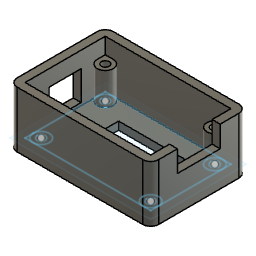
usb2uart (Autodesk Fusion 360 design; units mm, degrees)
Autodesk Fusion 360 part; units mm, degrees
sketch "Sketch1" plane through (0, 0, 0) normal (0, 1, 0) x (1, 0, 0)
  line L0 (0, 0) -> (53, 0)
  line L1 (53, 0) -> (53, -36)
  line L2 (53, -36) -> (0, -36)
  line L3 (0, -36) -> (0, 0)
  constraint horizontal L0
  constraint vertical L1
  constraint horizontal L2
  constraint vertical L3
  constraint coincident L0.start L3.end
extrude "Extrude1" add sketch "Sketch1" along normal blind 3
sketch "Sketch2" plane through (0, 3, 0) normal (0, 1, 0) x (-1, 0, 0)
  line L0 (0, 36) -> (-53, 36)
  line L1 (-53, 36) -> (-53, 0)
  line L2 (-53, 0) -> (0, 0)
  line L3 (0, 0) -> (0, 36)
  line L4 (-3, 3) -> (-50, 3)
  line L5 (-50, 3) -> (-50, 33)
  line L6 (-50, 33) -> (-3, 33)
  line L7 (-3, 33) -> (-3, 3)
  circle A0 centre (-47, 30) radius 3
  circle A1 centre (-47, 6) radius 3
  circle A2 centre (-6, 30) radius 3
  circle A3 centre (-6, 6) radius 3
  circle A4 centre (-6, 6) radius 1.5
  circle A5 centre (-6, 30) radius 1.5
  circle A6 centre (-47, 30) radius 1.5
  circle A7 centre (-47, 6) radius 1.5
  dimension "d3" = 6
  dimension "d4" = 6
  dimension "d5" = 3
  dimension "d6" = 3
  dimension "d7" = 3
  constraint horizontal L4
  constraint vertical L5
  constraint horizontal L6
  constraint vertical L7
  constraint tangent L7 A2
  constraint tangent L7 A3
  constraint concentric A3 A4
  constraint concentric A2 A5
  constraint concentric A0 A6
  constraint concentric A1 A7
  measures "d3" diameter of A1
  measures "d4" diameter of A2
  measures "d5" diameter of A4
  measures "d6" diameter of A5
  measures "d7" diameter of A6
extrude "Extrude2" add sketch "Sketch2" along normal blind 12 contours L4 L7 A3 | A3 | L4 L5 A1 | A1 | L6 L7 A2 | A2 | L5 L6 A0 | A0
extrude "Extrude3" add sketch "Sketch2" along normal blind 18 contours L0 L1 L2 L3
sketch "Sketch3" plane through (0, 0, 0) normal (-1, 0, 0) x (0, 0, 1)
  line L0 (0, 0) -> (36, 0)
  line L1 (36, 0) -> (36, 21)
  line L2 (36, 21) -> (0, 21)
  line L3 (0, 21) -> (0, 0)
  line L4 (12.0161, 21) -> (24.0161, 21)
  line L5 (24.0161, 21) -> (24.0161, 4)
  line L6 (24.0161, 4) -> (12.0161, 4)
  line L7 (12.0161, 4) -> (12.0161, 21)
  line L8 (12.0161, 21) -> (24.0161, 21)
  line L9 (24.0161, 21) -> (24.0161, 15)
  line L10 (24.0161, 15) -> (12.0161, 15)
  line L11 (12.0161, 15) -> (12.0161, 21)
  dimension "d12" = 12
  dimension "d13" = 17
  dimension "d14" = 6
  constraint horizontal L4
  constraint vertical L5
  constraint horizontal L6
  constraint vertical L7
  constraint coincident L2 L4.start
  constraint horizontal L8
  constraint vertical L9
  constraint horizontal L10
  constraint vertical L11
  measures "d12" distance of L4.start L4.end
  measures "d13" distance of L4.start L6.end
  measures "d14" distance of L4.start L10.end
extrude "Extrude4" cut sketch "Sketch3" against normal blind 11 contours L5 L6 L7 L10
sketch "Sketch4" plane through (53, 0, 0) normal (1, 0, 0) x (0, 0, -1)
  line L0 (-36, 0) -> (0, 0)
  line L1 (0, 0) -> (0, 21)
  line L2 (0, 21) -> (-36, 21)
  line L3 (-36, 21) -> (-36, 0)
  line L4 (-9.9926, 21) -> (-25.9926, 21)
  line L5 (-25.9926, 21) -> (-25.9926, 13)
  line L6 (-25.9926, 13) -> (-9.9926, 13)
  line L7 (-9.9926, 13) -> (-9.9926, 21)
  dimension "d17" = 16
  constraint horizontal L4
  constraint vertical L5
  constraint horizontal L6
  constraint vertical L7
  constraint coincident L2 L4.start
  measures "d17" distance of L4.start L4.end
extrude "Extrude5" cut sketch "Sketch4" against normal blind 6 contours L2 L4 L5 L6 L7
fillet "Fillet1" radius 3 1 edges at (53, 10.5, 0)
fillet "Fillet2" radius 3 1 edges at (0, 10.5, 0)
fillet "Fillet3" radius 3 1 edges at (0, 10.5, 36)
fillet "Fillet4" radius 3 1 edges at (53, 10.5, 36)
sketch "Sketch5" plane through (0, 0, 0) normal (0, -1, 0) x (1, 0, 0)
  arc A0 (53, 33) -> (50, 36) centre (50, 33) ccw
  line L0 (50, 36) -> (3, 36)
  arc A1 (3, 36) -> (0, 33) centre (3, 33) ccw
  line L1 (0, 33) -> (0, 3)
  arc A2 (0, 3) -> (3, 0) centre (3, 3) ccw
  line L2 (3, 0) -> (50, 0)
  arc A3 (50, 0) -> (53, 3) centre (50, 3) ccw
  line L3 (53, 3) -> (53, 33)
  line L4 (50, 10.0095) -> (15, 10.0095)
  line L5 (15, 10.0095) -> (15, 26.0095)
  line L6 (15, 26.0095) -> (50, 26.0095)
  line L7 (50, 26.0095) -> (50, 10.0095)
  line L8 (50, 10.0095) -> (45, 10.0095)
  line L9 (45, 10.0095) -> (45, 26.0095)
  line L10 (45, 26.0095) -> (50, 26.0095)
  line L11 (50, 26.0095) -> (50, 10.0095)
  dimension "d28" = 16
  dimension "d29" = 5
  constraint horizontal L4
  constraint vertical L5
  constraint horizontal L6
  constraint vertical L7
  constraint horizontal L8
  constraint vertical L9
  constraint horizontal L10
  constraint vertical L11
  measures "d28" distance of L4.start L6.end
  measures "d29" distance of L4.start L8.end
extrude "Extrude6" cut sketch "Sketch5" against normal blind 7 contours L4 L5 L6 L9
